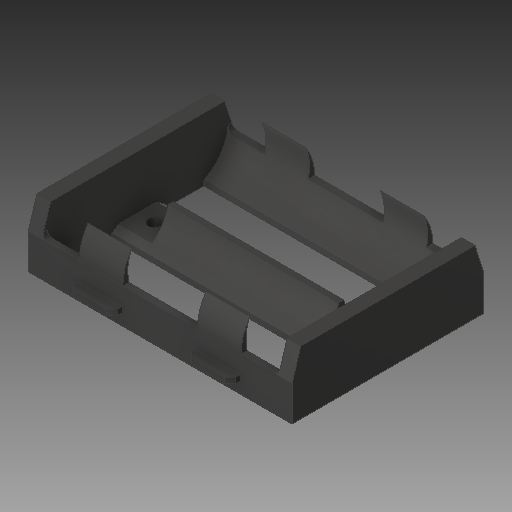
# Autodesk Inventor part: Keystone-26650-Dual-Battery-Holder[DWG-1109]
Saved by Autodesk Inventor 2017 (Build 210142000, 142)
## iProperties
Created: 2018-04-06
Part Number: Keystone-26650-Dual-Battery-Holder[DWG-1109]
Material: Thermoplastic Resin
Document SubType Name: Modeling
Designer: MtgSaber
Density: 1.28 g/cm^3
Appearance: Smooth - Black
Mass: 25.4413 g
Surface Area: 135.564 cm^2
Volume: 19.876 cm^3
Author: MtgSaber
Autodesk Inventor part; units mm, degrees
ref_plane "YZ Plane" through (0, 0, 0) normal (1, 0, 0) x (0, 1, 0)
sketch "Sketch1" plane through (0, 0, 0) normal (0, 1, 0) x (-1, 0, 0)
  line L0 (38.4302, 27.94) -> (-38.4302, 27.94)
  line L1 (-38.4302, 27.94) -> (-38.4302, -27.94)
  line L2 (-38.4302, -27.94) -> (38.4302, -27.94)
  line L3 (38.4302, -27.94) -> (38.4302, 27.94)
  line L4 (53.8023, 0) -> (-53.8023, 0) construction
  line L5 (0, -39.116) -> (0, 39.116) construction
  point P0 (0, 0)
  point P1 (0, 27.94)
  point P2 (38.4302, 0)
  dimension "d0" = 76.8604
  dimension "d1" = 55.88
  constraints: 8 end point, 2 midpoint, 2 parallel, 2 point on line, 1 horizontal, 1 perpendicular
  measures "d0" distance of L1.end L2.end
  measures "d1" distance of L0.end L1.end
extrude "Extrusion1" add sketch "Sketch1" along normal blind 18.415
ref_plane "Work Plane1" through (0, 0, 27.94) normal (1, 0, 0) x (0, 0, -1)
sketch "Sketch2" plane through (0, 0, 27.94) normal (1, 0, 0) x (0, 0, -1)
  line L0 (27.94, -6.8898) -> (27.94, 29.6482) construction
  line L1 (67.056, 0) -> (-11.176, 0) construction
  circle A0 centre (14.5034, 13.1588) radius 13.0493
  circle A1 centre (41.3766, 13.1588) radius 13.0493
  line L2 (1.8034, 10.16) -> (27.2034, 10.16) construction
  point P0 (27.94, 0)
  dimension "d4" = 13.4366
  dimension "d6" = 26.0985
  dimension "d11" = 25.4
  dimension "d12" = 10.16
  constraints: 2 centre point, 2 end point, 2 point on circle, 1 horizontal, 1 symmetric about line, 1 other
  measures "d4" distance from line of L0 A0.centre
  measures "d6" diameter of A0
  measures "d11" distance of L2.start L2.end
  measures "d12" distance between parallel lines of L1 L2
extrude "Extrusion2" cut sketch "Sketch2" along normal mid plane 68.961
sketch "Sketch3" plane through (-38.4302, 0, 27.94) normal (0, 0, 1) x (1, 0, 0)
  line L0 (0, 18.415) -> (76.8604, 18.415) construction
  line L1 (3.9497, 18.415) -> (3.9497, 0.1096) construction
  line L2 (3.9497, 18.415) -> (14.8717, 18.415)
  line L3 (14.8717, 18.415) -> (14.8717, 10.16)
  line L4 (14.8717, 10.16) -> (3.9497, 10.16)
  line L5 (3.9497, 10.16) -> (3.9497, 18.415)
  line L6 (27.5717, 18.415) -> (38.4302, 18.415)
  line L7 (27.5717, 10.16) -> (27.5717, 18.415)
  line L8 (-15.3721, 0) -> (92.2325, 0) construction
  line L9 (27.5717, 10.16) -> (38.4302, 10.16)
  line L10 (38.4302, -3.683) -> (38.4302, 22.098) construction
  line L11 (72.9107, 18.415) -> (61.9887, 18.415)
  line L12 (61.9887, 18.415) -> (61.9887, 10.16)
  line L13 (61.9887, 10.16) -> (72.9107, 10.16)
  line L14 (72.9107, 10.16) -> (72.9107, 18.415)
  line L15 (49.2887, 18.415) -> (38.4302, 18.415)
  line L16 (49.2887, 10.16) -> (49.2887, 18.415)
  line L17 (49.2887, 10.16) -> (38.4302, 10.16)
  point P0 (38.4302, 0)
  dimension "d13" = 10.922
  dimension "d16" = 10.16
  dimension "d17" = 12.7
  constraints: 28 end point, 6 symmetric about line, 3 horizontal, 3 parallel, 1 perpendicular, 1 point on line
  measures "d13" distance of L3.end L4.end
  measures "d16" distance between parallel lines of L8 L4
  measures "d17" distance between parallel lines of L7 L3
extrude "Extrusion3" cut sketch "Sketch3" against normal through all
sketch "Sketch4" plane through (-34.4805, 0, 27.94) normal (1, 0, 0) x (0, 0, -1)
  line L0 (27.2034, 10.16) -> (28.6766, 10.16) projected
  arc A0 (27.2034, 10.16) -> (26.4472, 18.415) centre (14.5034, 13.1588) ccw projected
  arc A1 (29.4328, 18.415) -> (28.6766, 10.16) centre (41.3766, 13.1588) ccw projected
  line L1 (29.4328, 18.415) -> (26.4472, 18.415) projected
  line L2 (0, 18.415) -> (2.5596, 18.415) projected
  arc A2 (2.5596, 18.415) -> (0, 10.16) centre (14.5917, 10.16) ccw
  line L3 (0, 18.415) -> (55.88, 18.415) construction
  line L4 (0, 10.16) -> (0, 18.415)
  line L5 (0, 18.415) -> (2.5596, 18.415)
  line L6 (27.94, -3.7218) -> (27.94, 22.3306) construction
  line L7 (55.88, 18.415) -> (53.3204, 18.415)
  arc A3 (55.88, 10.16) -> (53.3204, 18.415) centre (41.2883, 10.16) ccw
  line L8 (55.88, 10.16) -> (55.88, 18.415)
  line L9 (55.88, 18.415) -> (53.3204, 18.415)
  point P0 (27.94, 0)
  point P1 (0, 0)
  dimension "d21" = 14.5917
  constraints: 10 end point, 4 point on circle, 3 symmetric about line, 2 centre point, 1 perpendicular, 1 vertical, 1 other
  measures "d21" radius of A2
extrude "Extrusion4" cut sketch "Sketch4" along normal up to surface (68.961 mm away)
sketch "Sketch5" plane through (-34.4805, 0, 27.94) normal (1, 0, 0) x (0, 0, -1)
  arc A0 (1.8034, 10.16) -> (27.2034, 10.16) centre (14.5034, 13.1588) ccw construction
  arc A1 (28.6766, 10.16) -> (54.0766, 10.16) centre (41.3766, 13.1588) ccw construction
  line L0 (27.2034, 10.16) -> (28.6766, 10.16) projected
  line L1 (22.479, 2.8306) -> (33.401, 2.8306)
  arc A2 (22.479, 2.8306) -> (27.2034, 10.16) centre (14.5034, 13.1588) ccw
  arc A3 (28.6766, 10.16) -> (33.401, 2.8306) centre (41.3766, 13.1588) ccw
  point P0 (27.94, 0)
  dimension "d24" = 10.922
  constraints: 6 point on circle, 2 centre point, 2 concentric, 2 end point, 1 horizontal
  measures "d24" distance of L1.start L1.end
extrude "Extrusion5" cut sketch "Sketch5" along normal blind 9.652
mirror "Mirror1" about plane through (0, 0, 27.94) normal (1, 0, 0) of "Extrusion5"
sketch "Sketch6" plane through (-34.4805, 0, 27.94) normal (1, 0, 0) x (0, 0, -1)
  arc A0 (1.8034, 10.16) -> (22.479, 2.8306) centre (14.5034, 13.1588) ccw construction
  line L0 (55.88, 0) -> (0, 0) construction
  line L1 (8.6614, 1.4903) -> (8.6614, 0)
  line L2 (14.5034, 13.1588) -> (14.5034, 0) construction
  line L3 (20.3454, 1.4903) -> (20.3454, 0)
  arc A1 (8.6614, 1.4903) -> (20.3454, 1.4903) centre (14.5034, 13.1588) ccw
  line L4 (8.6614, 0) -> (20.3454, 0)
  point P0 (27.94, 0)
  dimension "d27" = 5.842
  constraints: 8 end point, 3 point on circle, 2 point on line, 2 symmetric about line, 1 centre point, 1 collinear, 1 concentric, 1 perpendicular, 1 vertical
  measures "d27" distance between parallel lines of L2 L1
extrude "Extrusion6" cut sketch "Sketch6" along normal up to surface (68.961 mm away)
ref_plane "Work Plane2" through (-38.4302, 0, 0) normal (0, 0, 1) x (1, 0, 0)
mirror "Mirror2" about plane through (-38.4302, 0, 0) normal (0, 0, 1) of "Extrusion6"
sketch "Sketch7" plane through (38.4302, 0, 27.94) normal (1, 0, 0) x (0, 0, -1)
  line L0 (0, 0) -> (0, 18.415) construction
  line L1 (0, 18.415) -> (55.88, 18.415) construction
  arc A0 (2.5596, 18.415) -> (0, 10.16) centre (14.5917, 10.16) ccw construction
  line L2 (2.5596, 18.415) -> (0, 10.16)
  line L3 (2.5596, 18.415) -> (0, 18.415)
  line L4 (0, 10.16) -> (0, 18.415)
  point P0 (27.94, 0)
  constraints: 6 end point, 1 collinear, 1 perpendicular, 1 tangent
extrude "Extrusion7" cut sketch "Sketch7" against normal up to surface (3.9497 mm away)
mirror "Mirror3" about plane through (-38.4302, 0, 0) normal (0, 0, 1) of "Extrusion7"
mirror "Mirror4" about plane through (0, 0, 27.94) normal (1, 0, 0) of "Extrusion7", "Mirror3"
fillet "Fillet1" radius 1.5875 4 edges at (-34.4805, 10.16, -27.0383) (-34.4805, 10.16, 27.0383) (34.4805, 10.16, -27.0383) (34.4805, 10.16, 27.0383)
sketch "Sketch9" plane through (-38.4302, 0, 27.94) normal (0, 0, 1) x (1, 0, 0)
  line L0 (27.5717, 10.16) -> (27.5717, 18.415) construction
  line L1 (14.8717, 18.415) -> (14.8717, 10.16) construction
  line L2 (0, 0) -> (76.8604, 0) construction
  line L3 (14.8717, 5.0927) -> (14.8717, 3.5052)
  line L4 (27.5717, 5.0927) -> (27.5717, 3.5052)
  line L5 (14.8717, 5.0927) -> (27.5717, 5.0927)
  line L6 (14.8717, 3.5052) -> (27.5717, 3.5052)
  point P0 (38.4302, 0)
  dimension "d33" = 3.5052
  dimension "d34" = 1.5875
  dimension "d36" = 12.7
  dimension "d37" = 12.7
  constraints: 8 end point, 4 perpendicular
  measures "d33" distance between parallel lines of L2 L6
  measures "d34" distance between parallel lines of L5 L6
  measures "d36" distance between parallel lines of L0 L3
  measures "d37" distance of L3.end L4.end
extrude "Extrusion8" add sketch "Sketch9" along normal blind 3.175
mirror "Mirror5" about plane through (0, 0, 27.94) normal (1, 0, 0) of "Extrusion8"
mirror "Mirror6" about plane through (-38.4302, 0, 0) normal (0, 0, 1) of "Extrusion8", "Mirror5"
chamfer "Chamfer1" distance 1.5875 angle 45 8 edges at (-10.8585, 4.299, 31.115) (23.5585, 4.2989, 31.115) (10.8585, 4.299, 31.115) (-23.5585, 4.2989, 31.115) (-10.8585, 4.299, -31.115) (-23.5585, 4.2989, -31.115) (23.5585, 4.2989, -31.115) (10.8585, 4.299, -31.115)
sketch "Sketch10" plane through (-34.4805, 2.8306, 5.461) normal (0, 1, 0) x (1, 0, 0)
  line L0 (-19.3218, 5.461) -> (88.2828, 5.461) construction
  line L1 (34.4805, 49.022) -> (34.4805, -38.1) construction
  point P0 (34.4805, 5.461)
  point P1 (4.8006, 5.461)
  dimension "d43" = 29.6799
  constraints: 1 point on line
  measures "d43" distance from line of L1 point (4.801, 5.461)
hole "Hole1" at (-29.6799, 2.8306, 0) direction (0, -1, 0) diameter 3.6576 end through all
mirror "Mirror7" about plane through (0, 0, 27.94) normal (1, 0, 0) of "Hole1"
body "Solid1"
